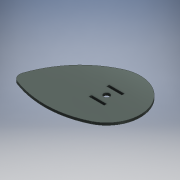
# Autodesk Inventor part: leva00
Saved by Autodesk Inventor 2016 (Build 200138000, 138)
## iProperties
Created: 2016-09-20
Part Number: leva00
Material: Madera (abedul)
Document SubType Name: Modeling
Designer: i95sa
Density: 0.55 g/cm^3
Appearance: Gris plomo - Pulido
Author: i95sa
Autodesk Inventor part; units mm, degrees
ref_plane "YZ Plane" through (0, 0, 0) normal (1, 0, 0) x (0, 1, 0)
ref_plane "XZ Plane" through (0, 0, 0) normal (0, 1, 0) x (-1, 0, 0)
ref_plane "XY Plane" through (0, 0, 0) normal (0, 0, 1) x (1, 0, 0)
sketch "Boceto1" plane through (0, 0, 0) normal (0, 0, 1) x (1, 0, 0)
  arc A0 (50.1681, 23.6073) -> (-50.1681, -23.6073) centre (0, 0) ccw
  arc A1 (-77.2048, -36.3298) -> (-100.3593, -47.2255) centre (-88.7821, -41.7777) ccw
  line L0 (-103.7113, -48.8028) -> (-109.1591, -37.2255)
  line L1 (-23.0114, 50.4443) -> (-32.0911, 69.7397)
  line L2 (-32.0911, 69.7397) -> (-109.1591, -37.2255)
  line L3 (-109.1591, -37.2255) -> (-79.2408, 4.299)
  arc A2 (-23.0114, 50.4443) -> (-79.2408, 4.299) centre (35.8738, -78.6405) ccw
  arc A3 (-79.2408, 4.299) -> (-100.8923, -37.648) centre (50.7496, -89.3585) ccw
  line L4 (3.8591, 1.8159) -> (50.1681, 23.6073)
  line L5 (-3.8591, -1.8159) -> (-103.7113, -48.8028)
  arc A4 (-50.1681, -23.6073) -> (50.1681, 23.6073) centre (0, 0) ccw
  arc A5 (-100.3593, -47.2255) -> (-77.2048, -36.3298) centre (-88.7821, -41.7777) ccw
  line L6 (-103.7113, -48.8028) -> (-98.2634, -60.3801)
  line L7 (24.2, -49.885) -> (33.2797, -69.1804)
  line L8 (33.2797, -69.1804) -> (-98.2634, -60.3801)
  line L9 (-98.2634, -60.3801) -> (-47.1976, -63.7964)
  arc A6 (-47.1976, -63.7964) -> (24.2, -49.885) centre (-37.7267, 77.7686) ccw
  arc A7 (-93.3195, -53.7411) -> (-47.1976, -63.7964) centre (-36.5029, 96.0625) ccw
  dimension "d0" = 110.89
  dimension "d6" = 25.59
  dimension "d7" = 12.795
  dimension "d8" = 21.325
  dimension "d9" = 51.18
  constraints: 20 end point, 20 point on circle, 8 centre point, 6 symmetric about line, 5 point on line, 4 tangent, 1 collinear, 4 other
  measures "d0" diameter of A0
  measures "d6" diameter of A1
  measures "d7" distance of L0.start L0.end
  measures "d8" distance of L1.start L1.end
  measures "d9" distance of L0.end L3.end
extrude "Extrusión2" add sketch "Boceto1" along normal blind 4 contours A4 A0 | A0 L5 A1 A3 A2 | A6 A7 A5 L5 A4 | L5 A1 | A5 L5
sketch "Boceto2" plane through (0, 0, 4) normal (0, 0, 1) x (1, 0, 0)
  line L0 (0, 0) -> (0, 12.5)
  line L1 (0, 12.5) -> (-12.5, 12.5)
  line L2 (-12.5, 12.5) -> (-12.5, 16.7)
  line L3 (-12.5, 16.7) -> (12.5, 16.7)
  line L4 (12.5, 16.7) -> (12.5, 12.5)
  line L5 (12.5, 12.5) -> (0, 12.5)
  line L6 (0, 0) -> (12.5, 0)
  line L7 (0, 0) -> (0, -12.5)
  line L8 (0, -12.5) -> (-12.5, -12.5)
  line L9 (-12.5, -12.5) -> (-12.5, -16.7)
  line L10 (-12.5, -16.7) -> (12.5, -16.7)
  line L11 (12.5, -16.7) -> (12.5, -12.5)
  line L12 (12.5, -12.5) -> (0, -12.5)
  circle A0 centre (0, 0) radius 5
  dimension "d24" = 12.5
  dimension "d25" = 12.5
  dimension "d26" = 4.2
  dimension "d27" = 25
  dimension "d28" = 10
  constraints: 26 end point, 5 perpendicular, 5 symmetric about line, 3 point on line, 1 centre point, 1 coincident, 1 parallel, 1 vertical
  measures "d24" distance of L0.start L0.end
  measures "d25" distance of L0.end L1.end
  measures "d26" distance of L1.end L2.end
  measures "d27" distance of L2.end L3.end
  measures "d28" diameter of A0
extrude "Extrusión3" cut sketch "Boceto2" against normal blind 4
